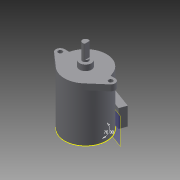
# Autodesk Inventor part: PG35L
Saved by Autodesk Inventor 2015 (Build 190159000, 159)
## iProperties
Created: 2014-01-21
Part Number: PG35L
Material: Generic
Document SubType Name: Modeling
Designer: Jack
Density: 1 g/cm^3
Appearance: Default
Author: Jack
Autodesk Inventor part; units mm, degrees
ref_plane "YZ Plane" through (0, 0, 0) normal (1, 0, 0) x (0, 1, 0)
ref_plane "XZ Plane" through (0, 0, 0) normal (0, 1, 0) x (-1, 0, 0)
ref_plane "XY Plane" through (0, 0, 0) normal (0, 0, 1) x (1, 0, 0)
sketch "Sketch1" plane through (0, 0, 0) normal (0, 0, 1) x (1, 0, 0)
  circle A0 centre (0, 0) radius 1.75
  circle A1 centre (42, 0) radius 1.75
  arc A2 (0, 3.65) -> (-2.4073, -2.7436) centre (0, 0) ccw
  arc A3 (44.4073, -2.7436) -> (42, 3.65) centre (42, 0) ccw
  line L0 (-2.4073, -2.7436) -> (9.4583, -13.1545)
  line L1 (32.5417, -13.1545) -> (44.4073, -2.7436)
  line L2 (42, 3.65) -> (38.1151, 3.65)
  line L3 (0, 3.65) -> (3.8849, 3.65)
  arc A4 (9.4583, -13.1545) -> (32.5417, -13.1545) centre (21, 0) ccw
  arc A5 (38.1151, 3.65) -> (3.8849, 3.65) centre (21, 0) ccw
  dimension "d0" = 3.5
  dimension "d2" = 42
  dimension "d3" = 7.3
  dimension "d5" = 21
  dimension "d6" = 17.5
  dimension "d7" = 17.5
  constraints: 8 end point, 8 point on circle, 6 centre point, 6 tangent, 3 coincident, 2 equal radius, 2 horizontal alignment, 1 collinear, 1 horizontal
  measures "d0" diameter of A0
  measures "d2" distance of A0.centre A1.centre
  measures "d3" diameter of A2
  measures "d5" distance of A1.centre A4.centre
  measures "d6" radius of A5
  measures "d7" radius of A4
extrude "Extrusion1" add sketch "Sketch1" along normal blind 5
sketch "Sketch2" plane through (0, 0, 5) normal (0, 0, 1) x (1, 0, 0)
  arc A0 (38.1151, 3.65) -> (3.8849, 3.65) centre (21, 0) ccw projected
  circle A1 centre (21, 0) radius 5
  dimension "d10" = 10
  constraints: 1 centre point, 1 coincident
  measures "d10" diameter of A1
extrude "Extrusion2" add sketch "Sketch2" along normal blind 4.7
sketch "Sketch3" plane through (21, 0, 9.7) normal (0, 0, 1) x (1, 0, 0)
  circle A0 centre (0, 0) radius 5 projected
  circle A1 centre (0, 0) radius 2.5
  point P0 (-21, 0)
  dimension "d13" = 5
  constraints: 1 centre point, 1 coincident
  measures "d13" diameter of A1
extrude "Extrusion3" add sketch "Sketch3" along normal blind 1.5 contours A1
sketch "Sketch4" plane through (21, 0, 11.2) normal (0, 0, 1) x (1, 0, 0)
  circle A0 centre (0, 0) radius 2.5 projected
  line L0 (1.5, 2) -> (1.5, -2)
  point P0 (-21, 0)
  dimension "d16" = 4
  constraints: 2 end point, 2 point on circle, 1 vertical
extrude "Extrusion4" add sketch "Sketch4" along normal blind 11.8 contours L0 A0 picked at (0.1918, -0.203)
sketch "Sketch5" plane through (0, 0, 0) normal (0, 0, -1) x (-1, 0, 0)
  arc A0 (-3.8849, 3.65) -> (-38.1151, 3.65) centre (-21, 0) ccw projected
  arc A1 (-32.5417, -13.1545) -> (-9.4583, -13.1545) centre (-21, 0) ccw projected
  circle A2 centre (-21, 0) radius 17.5
  constraints: 1 centre point, 1 coincident, 1 concentric
extrude "Extrusion5" add sketch "Sketch5" along normal blind 40
sketch "Sketch6" plane through (21, 0, -40) normal (0, 0, -1) x (-1, 0, 0)
  circle A0 centre (0, 0) radius 17.5 projected
  arc A1 (-1.5, -2) -> (-1.5, 2) centre (0, 0) ccw construction
  line L0 (0, 0) -> (-5.9854, 16.4446) construction
  circle A2 centre (21, 0) radius 1.75 construction
  line L1 (21, 0) -> (-17.5, 0) construction
  dimension "d21" = 70
  constraints: 4 end point, 2 point on circle, 1 horizontal
  measures "d21" angle of L1 L0
ref_plane "Work Plane1" through (26.9854, 16.4446, -40) normal (0.342, 0.9397, 0) x (-0.9397, 0.342, 0)
sketch "Sketch7" plane through (26.9854, 16.4446, -40) normal (0.342, 0.9397, 0) x (-0.9397, 0.342, 0)
  line L0 (-17.5, 0) -> (17.5, 0) projected
  line L1 (0, 0) -> (8.5, 0)
  line L2 (8.5, 0) -> (8.5, 15)
  line L3 (8.5, 15) -> (-8.5, 15)
  line L4 (-8.5, 15) -> (-8.5, 0)
  line L5 (-8.5, 0) -> (0, 0)
  point P0 (19.7335, 40)
  dimension "d22" = 8.5
  dimension "d23" = 15
  dimension "d24" = 17
  constraints: 10 end point, 2 perpendicular, 2 point on line, 1 collinear, 1 midpoint, 1 vertical
  measures "d22" distance of L1.start L1.end
  measures "d23" distance of L1.end L2.end
  measures "d24" distance of L2.end L3.end
extrude "Extrusion6" add sketch "Sketch7" along normal blind 6
body "Solid1"
